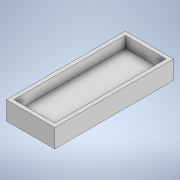
# Autodesk Inventor part: long-reed
Saved by Autodesk Inventor 2021 (Build 250183000, 183)
## iProperties
Created: 2021-01-17
Part Number: long-reed
Material: Generic
Document SubType Name: Modeling
Designer: Luke Kamols
Density: 1 g/cm^3
Appearance: Default
Author: Luke Kamols
Autodesk Inventor part; units mm, degrees
ref_plane "YZ Plane" through (0, 0, 0) normal (1, 0, 0) x (0, 1, 0)
ref_plane "XZ Plane" through (0, 0, 0) normal (0, 1, 0) x (-1, 0, 0)
ref_plane "XY Plane" through (0, 0, 0) normal (0, 0, 1) x (1, 0, 0)
sketch "Sketch1" plane through (0, 0, 0) normal (0, 1, 0) x (-1, 0, 0)
  line L0 (0, 0) -> (0, -32)
  line L1 (0, -32) -> (13, -32)
  line L2 (13, -32) -> (13, 0)
  line L3 (13, 0) -> (0, 0)
  dimension "d0" = 32
  dimension "d1" = 13
  constraints: 8 end point, 3 perpendicular, 1 vertical
  measures "d0" distance of L0.start L0.end
  measures "d1" distance of L0.end L1.end
extrude "Extrusion1" add sketch "Sketch1" along normal blind 2
sketch "Sketch2" plane through (0, 2, 0) normal (0, 1, 0) x (1, 0, 0)
  line L0 (-13, 32) -> (-13, 0) projected
  line L1 (0, 32) -> (-13, 32) projected
  line L2 (-13, 32) -> (-13, 0) projected
  line L3 (-13, 0) -> (0, 0) projected
  line L4 (0, 0) -> (0, 32) projected
  line L5 (0, 0) -> (0, 32) projected
  line L6 (0, 0) -> (0, 1)
  line L7 (-1, 1) -> (-12, 1)
  line L8 (-12, 1) -> (-12, 31)
  line L9 (-12, 31) -> (-1, 31)
  line L10 (-1, 31) -> (-1, 1)
  dimension "d5" = 1
  dimension "d6" = 11
  dimension "d7" = 30
  constraints: 10 end point, 2 parallel, 1 horizontal, 1 perpendicular, 1 point on line
  measures "d5" distance of L6.end L7.start
  measures "d6" distance of L8.end L9.end
  measures "d7" distance of L7.end L8.end
extrude "Extrusion2" add sketch "Sketch2" along normal blind 3
body "Solid1"
